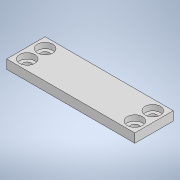
# Autodesk Inventor part: Крепление двигателя
Saved by Autodesk Inventor 2020 (Build 240168000, 168)
## iProperties
Created: 2021-06-13
Part Number: Крепление двигателя
Material: Типовые
Document SubType Name: Modeling
Designer: Антон
Density: 1 g/cm^3
Appearance: По умолчанию
Author: Антон
Autodesk Inventor part; units mm, degrees
ref_plane "YZ Plane" through (0, 0, 0) normal (1, 0, 0) x (0, 1, 0)
ref_plane "XZ Plane" through (0, 0, 0) normal (0, 1, 0) x (-1, 0, 0)
ref_plane "XY Plane" through (0, 0, 0) normal (0, 0, 1) x (1, 0, 0)
sketch "Эскиз1" plane through (0, 0, 0) normal (0, 1, 0) x (-1, 0, 0)
  line L0 (0, 0) -> (50, 0)
  line L1 (50, 0) -> (50, -15)
  line L2 (50, -15) -> (0, -15)
  line L3 (0, -15) -> (0, 0)
  dimension "d0" = 50
  dimension "d1" = 15
  constraints: 8 end point, 2 parallel, 1 horizontal, 1 perpendicular
  measures "d0" distance of L1.end L2.end
  measures "d1" distance of L0.end L1.end
extrude "Выдавливание1" add sketch "Эскиз1" along normal blind 3.5
sketch "Эскиз2" plane through (0, 3.5, 0) normal (0, 1, 0) x (1, 0, 0)
  line L0 (-50, 15) -> (-50, 0) projected
  line L1 (-50, 0) -> (-50, 4)
  line L2 (-50, 4) -> (-46, 4)
  line L3 (-50, 0) -> (0, 0) projected
  line L4 (-25, 0) -> (-25, 15)
  line L5 (0, 15) -> (-50, 15) projected
  line L6 (-50, 7.5) -> (0, 7.5)
  line L7 (0, 0) -> (0, 15) projected
  point P0 (-46, 11)
  point P1 (-4, 4)
  point P2 (-4, 11)
  dimension "d4" = 4
  constraints: 8 end point, 4 midpoint, 3 symmetric about line, 2 perpendicular, 1 point on line
  measures "d4" distance of L0.end L1.end
hole "Отверстие1" at (-46, 3.5, -4) at (-46, 3.5, -11) at (-4, 3.5, -11) at (-4, 3.5, -4) direction (0, -1, 0) diameter 3.2 end through all counterbore diameter 6 counterbore depth 2.15
